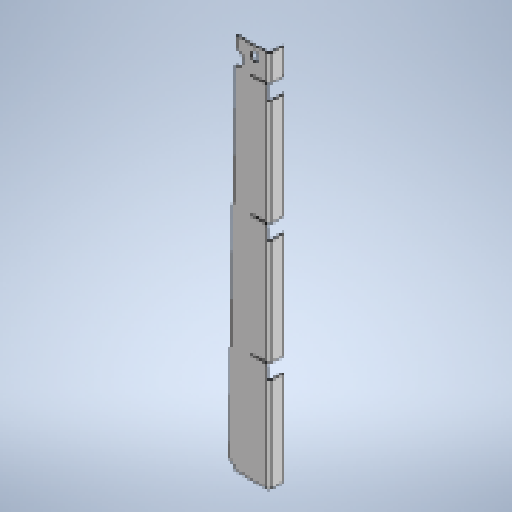
# Autodesk Inventor part: GBK 0201 second rib
Saved by Autodesk Inventor 2026.2 (Build 302298010, 298A)
## iProperties
Created: 2026-04-17
Part Number: GBK 0201 second rib
Material: Steel
Document SubType Name: Sheet Metal
Designer: pokla
Mass: 9630.75 g
Surface Area: 6306.22 cm^2
Volume: 1226.85 cm^3
Density: 7.85 g/cm^3
Sheet Metal Rule: Default
Appearance: Default
Flat Pattern Width: 22.343 cm
Flat Pattern Length: 156.361 cm
Flat Pattern Area: 3493.57 cm^2
Sheet Metal Width: 223,430 mm
Sheet Metal Length: 1563,606 mm
Sheet Metal Area: 349356,829 mm^2
Author: admin
Autodesk Inventor part; units mm, degrees
ref_plane "YZ Plane" through (0, 0, 0) normal (1, 0, 0) x (0, 1, 0)
ref_plane "XZ Plane" through (0, 0, 0) normal (0, 1, 0) x (-1, 0, 0)
ref_plane "XY Plane" through (0, 0, 0) normal (0, 0, 1) x (1, 0, 0)
sketch "Sketch1" plane through (0, 0, 0) normal (0, 0, 1) x (1, 0, 0)
  line L0 (0, 0) -> (0, 1479.6195)
  line L1 (0, 1479.6195) -> (-166.4399, 1479.6195)
  line L2 (-166.4399, 1479.6195) -> (-200, 0)
  line L3 (-200, 0) -> (0, 0)
  line L4 (0, 430) -> (-5, 430)
  line L5 (-5, 430) -> (-5, 368)
  line L6 (-5, 368) -> (0, 368)
  line L7 (0, 368) -> (0, 430)
  line L8 (-5, 430) -> (-70, 430)
  line L9 (-70, 430) -> (-70, 425)
  line L10 (-70, 425) -> (-5, 425)
  line L11 (-5, 425) -> (-5, 430)
  line L12 (-70, 430) -> (-190.2469, 430) construction
  line L13 (0, 4408.8661) -> (0, 1479.6195)
  line L14 (-166.4399, 1479.6195) -> (-132.8798, 2959.2389)
  line L15 (0, 4408.8661) -> (-100, 4408.8661)
  line L16 (-132.8798, 2959.2389) -> (0, 2959.2389)
  line L17 (-132.8798, 2959.2389) -> (-100, 4408.8661)
  line L18 (-5, 868) -> (0, 868)
  line L19 (-70, 925) -> (-5, 925)
  line L20 (-5, 930) -> (-70, 930)
  line L21 (-70, 930) -> (-70, 925)
  line L22 (-5, 925) -> (-5, 930)
  line L23 (-5, 930) -> (-5, 868)
  line L24 (0, 868) -> (0, 930)
  line L25 (0, 930) -> (-5, 930)
  line L26 (-5, 1368) -> (0, 1368)
  line L27 (-70, 1425) -> (-5, 1425)
  line L28 (-5, 1430) -> (-70, 1430)
  line L29 (-70, 1430) -> (-70, 1425)
  line L30 (-5, 1425) -> (-5, 1430)
  line L31 (-5, 1430) -> (-5, 1368)
  line L32 (0, 1368) -> (0, 1430)
  line L33 (0, 1430) -> (-5, 1430)
  line L34 (-5, 1868) -> (0, 1868)
  line L35 (-70, 1925) -> (-5, 1925)
  line L36 (-5, 1930) -> (-70, 1930)
  line L37 (-70, 1930) -> (-70, 1925)
  line L38 (-5, 1925) -> (-5, 1930)
  line L39 (-5, 1930) -> (-5, 1868)
  line L40 (0, 1868) -> (0, 1930)
  line L41 (0, 1930) -> (-5, 1930)
  line L42 (-5, 2368) -> (0, 2368)
  line L43 (-70, 2425) -> (-5, 2425)
  line L44 (-5, 2430) -> (-70, 2430)
  line L45 (-70, 2430) -> (-70, 2425)
  line L46 (-5, 2425) -> (-5, 2430)
  line L47 (-5, 2430) -> (-5, 2368)
  line L48 (0, 2368) -> (0, 2430)
  line L49 (0, 2430) -> (-5, 2430)
  line L50 (-5, 2868) -> (0, 2868)
  line L51 (-70, 2925) -> (-5, 2925)
  line L52 (-5, 2930) -> (-70, 2930)
  line L53 (-70, 2930) -> (-70, 2925)
  line L54 (-5, 2925) -> (-5, 2930)
  line L55 (-5, 2930) -> (-5, 2868)
  line L56 (0, 2868) -> (0, 2930)
  line L57 (0, 2930) -> (-5, 2930)
  line L58 (-100, 4408.8661) -> (-99.3197, 4438.8584) construction
  line L59 (0, 1629.6195) -> (-163.0377, 1629.6195)
  line L60 (-131.0653, 3039.2389) -> (0, 3039.2389)
  line L61 (-5, 3368) -> (0, 3368)
  line L62 (-70, 3425) -> (-5, 3425)
  line L63 (-5, 3430) -> (-70, 3430)
  line L64 (-70, 3430) -> (-70, 3425)
  line L65 (-5, 3425) -> (-5, 3430)
  line L66 (-5, 3430) -> (-5, 3368)
  line L67 (0, 3368) -> (0, 3430)
  line L68 (0, 3430) -> (-5, 3430)
  line L69 (-5, 3868) -> (0, 3868)
  line L70 (-70, 3925) -> (-5, 3925)
  line L71 (-5, 3930) -> (-70, 3930)
  line L72 (-70, 3930) -> (-70, 3925)
  line L73 (-5, 3925) -> (-5, 3930)
  line L74 (-5, 3930) -> (-5, 3868)
  line L75 (0, 3868) -> (0, 3930)
  line L76 (0, 3930) -> (-5, 3930)
  arc A0 (-140, 0) -> (-198.6395, 59.9846) centre (-200, 0) ccw
  arc A1 (-167.1202, 1449.6272) -> (-165.7596, 1509.6117) centre (-166.4399, 1479.6195) ccw
  arc A2 (-133.5601, 2929.2466) -> (-132.1995, 2989.2312) centre (-132.8798, 2959.2389) ccw
  line L77 (0, 930) -> (-70, 930)
  line L78 (-70, 930) -> (-178.9061, 930) construction
  line L79 (-70, 1430) -> (-167.5654, 1430) construction
  line L80 (-70, 1930) -> (-156.2246, 1930) construction
  line L81 (-70, 2430) -> (-144.8838, 2430) construction
  line L82 (-70, 2930) -> (-133.543, 2930) construction
  line L83 (-70, 3430) -> (-122.2022, 3430) construction
  line L84 (-70, 3930) -> (-110.8614, 3930) construction
  line L85 (-54.8875, 3005.2389) -> (-54.8875, 2995.2389) construction
  line L86 (-68.8875, 3005.2389) -> (-68.8875, 2995.2389)
  line L87 (-40.8875, 2995.2389) -> (-40.8875, 3005.2389)
  arc A3 (-40.8875, 3005.2389) -> (-68.8875, 3005.2389) centre (-54.8875, 3005.2389) ccw
  arc A4 (-68.8875, 2995.2389) -> (-40.8875, 2995.2389) centre (-54.8875, 2995.2389) ccw
  point P0 (0, 430)
  point P1 (-136.4399, 1479.6195)
  point P2 (-54.8875, 3000.2389)
  point P3 (-102.8875, 2958.5586)
  point P4 (-54.8875, 2981.2389)
  point P5 (-54.8875, 3019.2389)
  dimension "d25" = 430
  dimension "d32" = 1480
  dimension "d33" = 1480
  dimension "d34" = 1450
  dimension "d35" = 100
  dimension "d38" = 500
  dimension "d44" = 30
  dimension "d45" = 150
  dimension "d46" = 80
  dimension "d47" = 200
  dimension "d48" = 5
  dimension "d50" = 62
  dimension "d51" = 60
  dimension "d52" = 30
  dimension "d53" = 478.8661
  dimension "d54" = 30
  dimension "d56" = 190.2469
  dimension "d57" = 178.9061
  dimension "d58" = 167.5654
  dimension "d59" = 156.2246
  dimension "d60" = 144.8838
  dimension "d61" = 133.543
  dimension "d62" = 122.2022
  dimension "d63" = 110.8614
  dimension "d64" = 70
  dimension "d66" = 48
  dimension "d67" = 28
  dimension "d68" = 38
  dimension "d69" = 20
  measures "d25" distance between parallel lines of L3 L8
  measures "d32" distance of L2.end L1.end
  measures "d33" distance of L1.end L14.end
  measures "d34" distance of L14.end L15.end
  measures "d35" distance of L13.start L15.end
  measures "d38" distance of L6.start L18.start
  measures "d44" distance of L15.end L58.end
  measures "d45" distance between parallel lines of L1 L59
  measures "d46" distance between parallel lines of L16 L60
  measures "d47" distance of L2.end L0.start
  measures "d48" distance between parallel lines of L10 L8
  measures "d50" distance of L8.start L6.start
  measures "d51" radius of A0
  measures "d52" radius of A1
  measures "d53" distance from line of L71 L13.start
  measures "d54" radius of A2
  measures "d56" distance of L12.end L4.start
  measures "d57" distance of L78.end L24.end
  measures "d58" distance of L79.end L32.end
  measures "d59" distance of L80.end L40.end
  measures "d60" distance of L81.end L48.end
  measures "d61" distance of L82.end L56.end
  measures "d62" distance of L83.end L67.end
  measures "d63" distance of L84.end L75.end
  measures "d64" distance between parallel lines of L9 L0
  measures "d66" distance from line of point (-102.888, 2958.559) L85
  measures "d67" distance between parallel lines of L86 L87
  measures "d68" distance of point (-54.888, 2981.239) point (-54.888, 3019.239)
  measures "d69" distance from line of point (-54.888, 3019.239) L60
extrude "Plate1" add sketch "Sketch1" along normal blind 4 contours A1 L14 L59 L13 L1 | L14 A2 L16 L13 L57 L52 L53 L51 L55 L50 L49 L44 L45 L43 L47 L42 L41 L36 L37 L35 L39 L34 L59 | A2 L17 L60 L13 L16
sketch "Sketch2" plane through (4, 1479.6195, 4) normal (-1, 0, 0) x (0, -1, 0)
  line L0 (-388.3805, 0) -> (0, 0)
  line L1 (0, 0) -> (0, -60)
  line L2 (0, -60) -> (-388.3805, -60)
  line L3 (-388.3805, -60) -> (-388.3805, 0)
  constraints: 8 end point
edge flange "Flange1" height 60 angle 90 thickness 4 bend radius 4 thickness toward (-1, 0, 0) relief straight relief width 4 relief depth 2 corner gap 4 corner form 0 edges at (0, 1673.8097, 0) (0, 2149, 0) (0, 2649, 0) (0, 2984.6195, 0) wall of the first edge with corners at (4, 1868, 4) (4, 1479.6195, 4) (4, 1479.6195, -56) (4, 1868, -56)
bend "Bend1"
corner "Corner1"
chamfer "Corner Chamfer1" distance 10 angle 45 3 edges at (-5, 1925, 2) (-5, 2425, 2) (-5, 2925, 2)
equation "\"d5\" = Thickness"
equation "\"d7\" = BendReliefWidth"
equation "\"d8\" = BendReliefDepth"
equation "\"d9\" = MinimumRemnant"
equation "\"d10\" = TransitionRadius"
equation "\"d13\" = BendRadius"
equation "\"d14\" = CornerReliefSize"
equation "\"d15\" = GapSize"
equation "\"d16\" = JacobiRadiusSize"
equation "\"BendRadius\" = Thickness"
equation "\"BendReliefWidth\" = Thickness"
equation "\"BendReliefDepth\" = 0.5 * Thickness"
equation "\"CornerReliefSize\" = 4 * Thickness"
equation "\"MinimumRemnant\" = 2 * Thickness"
equation "\"TransitionRadius\" = BendRadius"
equation "\"JacobiRadiusSize\" = BendRadius"
equation "\"GapSize\" = Thickness"
equation "\"Thickness\" = 4"
body "Solid1"
